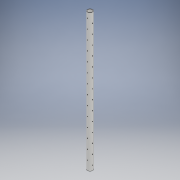
# Autodesk Inventor part: Ground_Antenna700mm_Support
Saved by Autodesk Inventor 2018 (Build 220112000, 112)
## iProperties
Created: 2018-10-12
Part Number: Ground_Antenna700mm_Support
Material: PVC-Piping
Document SubType Name: Modeling
Designer: Bradley
Density: 1.4 g/cm^3
Appearance: Smooth - White
Mass: 594.901 g
Surface Area: 2131.77 cm^2
Volume: 424.929 cm^3
Author: Bradley
Autodesk Inventor part; units mm, degrees
ref_plane "YZ Plane" through (0, 0, 0) normal (1, 0, 0) x (0, 1, 0)
ref_plane "XZ Plane" through (0, 0, 0) normal (0, 1, 0) x (-1, 0, 0)
ref_plane "XY Plane" through (0, 0, 0) normal (0, 0, 1) x (1, 0, 0)
sketch "Sketch1" plane through (0, 0, 0) normal (0, 0, 1) x (1, 0, 0)
  circle A0 centre (0, 0) radius 21.082
  circle A1 centre (0, 0) radius 17.526
  dimension "d0" = 42.164
  dimension "d1" = 35.052
  constraints: 2 centre point, 2 coincident
  measures "d0" diameter of A0
  measures "d1" diameter of A1
extrude "Extrusion1" add sketch "Sketch1" along normal mid plane 1150
sketch "Sketch3" plane through (0, 0, 0) normal (1, 0, 0) x (0, 1, 0)
  line L0 (-21.082, -575) -> (-21.082, 575) projected
  line L1 (17.526, -575) -> (-17.526, -575) projected
  point P0 (0, 0)
  point P1 (0, -535.7917)
  point P2 (0, -575)
  point P3 (0, -456.4918)
  point P4 (0, -377.1918)
  point P5 (0, -297.8918)
  point P6 (0, -218.5917)
  point P7 (0, -139.2918)
  point P8 (0, -59.9918)
  point P9 (0, 19.3082)
  point P10 (0, 98.6082)
  point P11 (0, 177.9082)
  point P12 (0, 257.2082)
  point P13 (0, 336.5082)
  point P14 (0, 415.8082)
  point P15 (0, 495.1082)
  dimension "d19" = 39.2082
  dimension "d22" = 79.3
  constraints: 1 midpoint, 1 vertical, 1 vertical alignment, 13 other
  measures "d19" distance from line of L1 point (0, -535.792)
  measures "d22" distance of point (0, -535.792) point (0, -456.492)
hole "Hole2" at (0, 0, -535.7917) at (0, 0, -456.4918) at (0, 0, -377.1918) at (0, 0, -297.8918) at (0, 0, -218.5917) at (0, 0, -139.2918) at (0, 0, -59.9918) at (0, 0, 19.3082) at (0, 0, 98.6082) at (0, 0, 177.9082) at (0, 0, 257.2082) at (0, 0, 336.5082) at (0, 0, 415.8082) at (0, 0, 495.1082) direction (-1, 0, 0) diameter 6.35 end through all both
sketch "Sketch4" plane through (0, 0, 0) normal (0, 1, 0) x (-1, 0, 0)
  line L0 (21.082, -538.9668) -> (17.526, -538.9668) projected
  line L1 (-17.526, -459.6668) -> (-21.082, -459.6668) projected
  line L2 (-17.526, -459.6668) -> (17.526, -538.9668) construction
  line L3 (-21.082, -575) -> (-21.082, 575) projected
  point P0 (0, 0)
  point P1 (0, -499.3167)
  point P2 (0, -420.0168)
  point P3 (0, -340.7167)
  point P4 (0, -261.4167)
  point P5 (0, -182.1167)
  point P6 (0, -102.8167)
  point P7 (0, -23.5168)
  point P8 (0, 55.7832)
  point P9 (0, 135.0832)
  point P10 (0, 214.3832)
  point P11 (0, 293.6832)
  point P12 (0, 372.9832)
  point P13 (0, 452.2832)
  point P14 (0, 531.5833)
  dimension "d36" = 79.3
  constraints: 2 end point, 1 midpoint, 1 vertical, 13 other
  measures "d36" distance of point (0, -499.317) point (0, -420.017)
hole "Hole3" at (0, 0, -499.3167) at (0, 0, -420.0168) at (0, 0, -340.7167) at (0, 0, -261.4167) at (0, 0, -182.1167) at (0, 0, -102.8167) at (0, 0, -23.5168) at (0, 0, 55.7832) at (0, 0, 135.0832) at (0, 0, 214.3832) at (0, 0, 293.6832) at (0, 0, 372.9832) at (0, 0, 452.2832) at (0, 0, 531.5833) direction (0, -1, 0) diameter 6.35 end through all both
equation "\"d36\" = d22"
body "Solid1"
